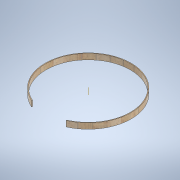
# Autodesk Inventor part: Banding Mid Level Inner
Saved by Autodesk Inventor 2020 (Build 240168000, 168)
## iProperties
Created: 2020-03-10
Part Number: Banding Mid Level Inner
Material: Wood (Maple)
Document SubType Name: Sheet Metal
Designer: Daniel Wikman
Density: 0.67 g/cm^3
Sheet Metal Rule: Default_mm
Appearance: Natural Maple - Glossy Dark Tint
Author: Daniel Wikman
Autodesk Inventor part; units mm, degrees
ref_plane "YZ Plane" through (0, 0, 0) normal (1, 0, 0) x (0, 1, 0)
ref_plane "XZ Plane" through (0, 0, 0) normal (0, 1, 0) x (-1, 0, 0)
ref_plane "XY Plane" through (0, 0, 0) normal (0, 0, 1) x (1, 0, 0)
sketch "Sketch1" plane through (0, 0, 0) normal (0, 1, 0) x (-1, 0, 0)
  circle A0 centre (0, 0) radius 233.71
  circle A1 centre (0, 0) radius 229.71
  dimension "d84" = 459.42
  dimension "d85" = 467.42
  constraints: 2 centre point, 1 coincident
  measures "d84" diameter of A1
  measures "d85" diameter of A0
extrude "Extrusion3" add sketch "Sketch1" along normal blind 30
sketch "Sketch3" plane through (0, 30, 0) normal (0, 1, 0) x (1, 0, 0)
  arc A0 (-132.1078, -408.1526) -> (132.1134, -408.1508) centre (0, 0) ccw
  arc A1 (-77.7244, -128.3741) -> (77.7297, -128.3709) centre (0, 0) ccw
  line L0 (-122.1811, -173.696) -> (-161.3589, -227.6196)
  line L1 (-132.1078, -408.1526) -> (-77.7244, -128.3741)
  line L2 (0, 0) -> (0, -341.2918)
  line L3 (132.1134, -408.1508) -> (77.7297, -128.3709)
  line L4 (210.5535, -295.3313) -> (171.3679, -241.3969) projected
  dimension "d52" = 25
  dimension "d87" = 150.07
  dimension "d88" = 429
  dimension "d89" = 25
  dimension "d90" = 11
  dimension "d91" = 11
  constraints: 8 end point, 4 point on circle, 2 centre point, 1 coincident, 2 other
  measures "d52" angle of L0 L1
  measures "d87" radius of A1
  measures "d88" radius of A0
  measures "d89" angle of L4 L3
  measures "d90" angle of L3 L2
  measures "d91" angle of L1 L2
extrude "Extrusion10" cut sketch "Sketch3" against normal through all
equation "\"BendRadius\" = Thickness"
equation "\"BendReliefWidth\" = Thickness"
equation "\"BendReliefDepth\" = 0.5 * Thickness"
equation "\"CornerReliefSize\" = 4 * Thickness"
equation "\"MinimumRemnant\" = 2 * Thickness"
equation "\"TransitionRadius\" = BendRadius"
equation "\"JacobiRadiusSize\" = BendRadius"
equation "\"GapSize\" = Thickness"
equation "\"Thickness\" = 0.5"
body "Solid3"
